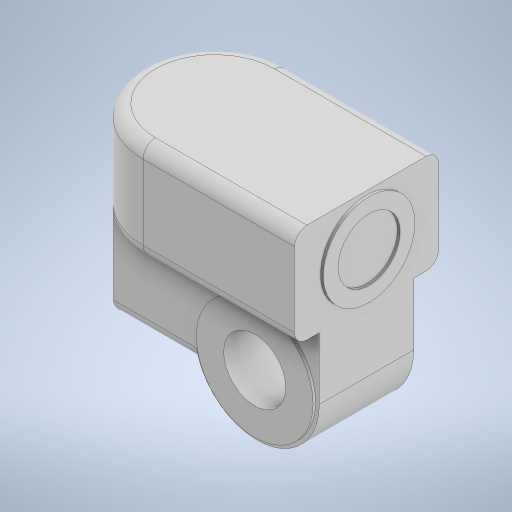
# Autodesk Inventor part: part3
Saved by Autodesk Inventor 2024.1 (Build 281209000, 209)
## iProperties
Created: 2023-08-22
Part Number: part3
Material: Generic
Document SubType Name: Modeling
Designer: admins
Density: 1 g/cm^3
Appearance: Default
Author: admins
Autodesk Inventor part; units mm, degrees
ref_plane "YZ Plane" through (0, 0, 0) normal (1, 0, 0) x (0, 1, 0)
ref_plane "XZ Plane" through (0, 0, 0) normal (0, 1, 0) x (-1, 0, 0)
ref_plane "XY Plane" through (0, 0, 0) normal (0, 0, 1) x (1, 0, 0)
sketch "Sketch1" plane through (0, 0, 0) normal (0, 1, 0) x (-1, 0, 0)
  line L0 (221.2262, 97.1913) -> (41.2262, 97.1913)
  line L1 (41.2262, 97.1913) -> (41.2262, 213.1913)
  line L2 (41.2262, 213.1913) -> (221.2262, 213.1913)
  line L3 (221.2262, 213.1913) -> (221.2262, 97.1913)
  point P0 (0, 0)
  dimension "d2" = 180
  dimension "d3" = 116
  constraints: 8 end point, 2 parallel, 1 horizontal, 1 perpendicular
  measures "d2" distance of L1.end L2.end
  measures "d3" distance of L0.end L1.end
extrude "Extrusion1" add sketch "Sketch1" along normal blind 180
sketch "Sketch2" plane through (-41.2262, 0, 97.1913) normal (0, 0, -1) x (-1, 0, 0)
  point P0 (-41.2262, 0)
sketch "Sketch3" plane through (-41.2262, 0, 213.1913) normal (1, 0, 0) x (0, 0, -1)
  line L0 (0, 0) -> (20, 0)
  line L1 (0, 0) -> (116, 0) projected
  line L2 (20, 0) -> (96, 0)
  line L3 (20, 0) -> (0, 0)
  line L4 (0, 0) -> (0, 100)
  line L5 (0, 100) -> (20, 100)
  line L6 (20, 100) -> (20, 0)
  line L7 (96, 0) -> (116, 0)
  line L8 (116, 0) -> (116, 100)
  line L9 (116, 100) -> (96, 100)
  line L10 (96, 100) -> (96, 0)
  point P0 (213.1913, 0)
  dimension "d6" = 20
  dimension "d7" = 76
  dimension "d8" = 20
  dimension "d9" = 100
  dimension "d10" = 20
  dimension "d11" = 100
  constraints: 20 end point, 4 parallel, 2 horizontal, 2 perpendicular, 2 point on line
  measures "d6" distance of L0.start L0.end
  measures "d7" distance of L0.end L2.end
  measures "d8" distance of L4.end L5.end
  measures "d9" distance of L3.end L4.end
  measures "d10" distance of L9.end L8.end
  measures "d11" distance of L8.end L7.end
extrude "Extrusion2" cut sketch "Sketch3" against normal blind 200 contours L4 L5 L6 L0
extrude "Extrusion3" cut sketch "Sketch3" against normal blind 200 contours L10 L9 L8 L1
sketch "Sketch4" plane through (-41.2262, 0, 117.1913) normal (0, 0, -1) x (-1, 0, 0)
  circle A0 centre (50, 50) radius 50
  line L0 (180, 0) -> (0, 0) projected
  line L1 (0, 0) -> (0, 100) projected
  circle A1 centre (50, 50) radius 47
  line L2 (180, 0) -> (180, 30)
  line L3 (180, 0) -> (180, 100) projected
  line L4 (180, 30) -> (95.8258, 30)
  point P0 (-41.2262, 0)
  point P1 (0, 50)
  point P2 (50, 0)
  dimension "d16" = 100
  dimension "d17" = 94
  dimension "d29" = 30
  constraints: 4 end point, 1 centre point, 1 coincident, 1 horizontal, 1 perpendicular, 1 point on line, 1 vertical, 3 other
  measures "d17" diameter of A1
  measures "d29" distance of L0.start L2.end
extrude "Extrusion4" add sketch "Sketch4" along normal blind 2 contours A1
sketch "Sketch5" plane through (-41.2262, 0, 193.1913) normal (0, 0, 1) x (1, 0, 0)
  circle A0 centre (-50, 50) radius 50
  line L0 (0, 100) -> (0, 0) projected
  line L1 (0, 0) -> (-180, 0) projected
  circle A1 centre (-50, 50) radius 47
  point P0 (41.2262, 0)
  dimension "d20" = 100
  dimension "d21" = 94
  constraints: 2 centre point, 2 tangent, 1 coincident
  measures "d20" diameter of A0
  measures "d21" diameter of A1
extrude "Extrusion5" add sketch "Sketch5" along normal blind 2 contours A1
sketch "Sketch6" plane through (-91.2262, 50, 115.1913) normal (0, 0, -1) x (-1, 0, 0)
  circle A0 centre (0, 0) radius 25
  point P0 (-91.2262, -50)
  dimension "d24" = 50
  constraints: 1 centre point
  measures "d24" diameter of A0
extrude "Extrusion6" cut sketch "Sketch6" against normal blind 200
extrude "Extrusion7" cut sketch "Sketch4" against normal blind 200 contours L0 L1 A0
sketch "Sketch7" plane through (-41.2262, 100, 117.1913) normal (0, 0, -1) x (-1, 0, 0)
  point P0 (-41.2262, -100)
extrude "Extrusion8" cut sketch "Sketch4" against normal blind 200 contours L4 L2 L0 A0
sketch "Sketch8" plane through (0, 180, 0) normal (0, 1, 0) x (1, 0, 0)
  circle A0 centre (-163.2262, -155.1913) radius 58
  line L0 (-221.2262, -97.1913) -> (-221.2262, -213.1913) projected
  line L1 (-221.2262, -213.1913) -> (-41.2262, -213.1913) projected
  line L2 (-41.2262, -213.1913) -> (-41.2262, -97.1913) projected
  line L3 (-221.2262, -213.1913) -> (-41.2262, -213.1913)
  line L4 (-41.2262, -213.1913) -> (-41.2262, -97.1913)
  line L5 (-221.2262, -97.1913) -> (-221.2262, -213.1913)
  line L6 (-221.2262, -97.1913) -> (-41.2262, -97.1913)
  line L7 (-221.2262, -97.1913) -> (-221.2262, -117.1913) projected
  point P0 (0, 0)
  point P1 (-163.2262, -97.1913)
  point P2 (-221.2262, -155.1913)
  point P3 (-163.2262, -213.1913)
  dimension "d32" = 116
  constraints: 8 end point, 2 perpendicular, 2 tangent, 1 centre point, 1 horizontal, 1 parallel
  measures "d32" diameter of A0
extrude "Extrusion9" cut sketch "Sketch8" against normal blind 200 contours A0 L0 L6
extrude "Extrusion10" cut sketch "Sketch8" against normal blind 200 contours L1 L0 A0
sketch "Sketch10" plane through (-41.2262, 180, 213.1913) normal (1, 0, 0) x (0, 0, -1)
  circle A0 centre (58, -40) radius 37
  circle A1 centre (58, -40) radius 25
  point P0 (213.1913, -180)
  dimension "d39" = 74
  dimension "d40" = 50
  constraints: 2 centre point, 1 coincident
  measures "d39" diameter of A0
  measures "d40" diameter of A1
extrude "Extrusion11" add sketch "Sketch10" along normal blind 2
fillet "Fillet2" radius 10 2 edges at (-187.3094, 100, 102.4277) (-102.2262, 100, 97.1913)
fillet "Fillet3" radius 10 7 edges at (-102.2262, 100, 213.1913) (-102.2262, 180, 213.1913) (-102.2262, 180, 97.1913) (-221.2262, 180, 155.1913) (-221.2262, 30, 155.1913) (-172.048, 30, 117.1913) (-172.048, 30, 193.1913)
body "Solid1"
